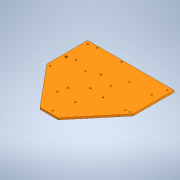
# Autodesk Inventor part: bp_v2
Saved by Autodesk Inventor 2020.3 (Build 243373000, 373)
## iProperties
Created: 2020-06-30
Part Number: bp_v2
Material: PET Plastic
Document SubType Name: Modeling
Designer: Devin
Density: 1.541 g/cm^3
Appearance: Orange
Author: Devin
Autodesk Inventor part; units mm, degrees
ref_plane "YZ Plane" through (0, 0, 0) normal (1, 0, 0) x (0, 1, 0)
ref_plane "XZ Plane" through (0, 0, 0) normal (0, 1, 0) x (-1, 0, 0)
ref_plane "XY Plane" through (0, 0, 0) normal (0, 0, 1) x (1, 0, 0)
sketch "Sketch1" plane through (0, 0, 0) normal (0, 1, 0) x (-1, 0, 0)
  line L0 (0, 0) -> (-190, 0)
  line L1 (-95, 180) -> (-75, 180)
  line L2 (-75, 180) -> (0, 90)
  line L3 (-95, 180) -> (-115, 180)
  line L4 (-115, 180) -> (-190, 90)
  line L5 (0, 0) -> (0, 90)
  line L6 (-190, 0) -> (-190, 90)
  dimension "d1" = 190
  dimension "d39" = 20
  dimension "d40" = 20
  constraints: 14 end point, 3 horizontal, 1 parallel, 1 vertical
  measures "d1" distance of L0.start L0.end
  measures "d39" distance of L1.start L1.end
  measures "d40" distance of L1.start L3.end
extrude "Extrusion1" add sketch "Sketch1" along normal blind 4
sketch "Sketch14" plane through (0, 4, 0) normal (0, 1, 0) x (1, 0, 0)
  line L0 (190, 0) -> (0, 0) projected
  line L1 (0, 0) -> (0, -7.5)
  line L2 (0, 0) -> (0, -15) projected
  line L3 (0, -90) -> (75, -180) projected
  circle A0 centre (7.5, -7.5) radius 1.55
  circle A1 centre (7.5, -90) radius 1.55
  line L4 (75, -180) -> (115, -180) projected
  circle A2 centre (182.5, -7.5) radius 1.55
  circle A3 centre (182.5, -90) radius 1.55
  circle A4 centre (95, -172.5) radius 1.55
  dimension "d68" = 7.5
  dimension "d71" = 3.1
  dimension "d72" = 3.1
  dimension "d74" = 3.1
  constraints: 5 centre point, 2 end point, 1 midpoint
  measures "d68" distance of L0.end L1.end
  measures "d71" diameter of A0
  measures "d72" diameter of A1
  measures "d74" diameter of A4
extrude "Extrusion10" cut sketch "Sketch14" against normal blind 10
sketch "Sketch17" plane through (0, 4, 0) normal (0, 1, 0) x (1, 0, 0)
  line L0 (93.28, -54.34) -> (12, -54.34)
  line L1 (12, -54.34) -> (12, -1)
  line L2 (12, -1) -> (93.28, -1)
  line L3 (93.28, -1) -> (93.28, -54.34)
  line L4 (93.28, -54.34) -> (93.28, -50.7586)
  circle A0 centre (79.5513, -50.7586) radius 1.55
  circle A1 centre (24.6238, -50.7586) radius 1.55
  line L5 (93.28, -1) -> (93.28, -3.8194)
  circle A2 centre (78.3321, -3.8194) radius 1.55
  circle A3 centre (24.6238, -3.8194) radius 1.55
  point P0 (0, 0)
  dimension "d101" = 81.28
  dimension "d102" = 53.34
  dimension "d106" = 3.1
  dimension "d107" = 3.1
  dimension "d111" = 3.1
  dimension "d112" = 3.1
  dimension "d113" = 14.9479
  dimension "d114" = 2.8194
  dimension "d115" = 12.6238
  dimension "d116" = 2.8194
  dimension "d117" = 12.6238
  dimension "d118" = 3.5814
  dimension "d119" = 3.5814
  dimension "d120" = 13.7287
  constraints: 12 end point, 4 centre point, 2 parallel, 2 point on line, 1 perpendicular
  measures "d101" distance of L0.start L0.end
  measures "d102" distance of L0.end L1.end
  measures "d106" diameter of A0
  measures "d107" diameter of A1
  measures "d111" diameter of A2
  measures "d112" diameter of A3
  measures "d113" distance from line of L3 A2.centre
  measures "d114" distance from line of L2 A2.centre
  measures "d115" distance from line of L1 A3.centre
  measures "d116" distance from line of L2 A3.centre
  measures "d117" distance from line of L1 A1.centre
  measures "d118" distance from line of L0 A1.centre
  measures "d119" distance from line of L0 A0.centre
  measures "d120" distance from line of L3 A0.centre
sketch "Sketch18" plane through (0, 4, 0) normal (0, 1, 0) x (1, 0, 0)
  line L0 (190, 0) -> (0, 0) projected
  line L1 (190, -90) -> (190, 0) projected
  line L2 (175, -10) -> (125, -10)
  line L3 (122, -13) -> (122, -92)
  line L4 (125, -95) -> (175, -95)
  line L5 (178, -92) -> (178, -13)
  circle A0 centre (174.5, -91.5) radius 1.375
  circle A1 centre (125.5, -91.5) radius 1.4481
  circle A2 centre (125.5, -33.5) radius 1.375
  circle A3 centre (174.5, -33.5) radius 1.375
  arc A4 (125, -10) -> (122, -13) centre (125, -13) ccw
  arc A5 (178, -13) -> (175, -10) centre (175, -13) ccw
  arc A6 (175, -95) -> (178, -92) centre (175, -92) ccw
  arc A7 (122, -92) -> (125, -95) centre (125, -92) ccw
  point P0 (122, -10)
  dimension "d129" = 2.75
  dimension "d130" = 3.5
  dimension "d131" = 3.5
  dimension "d132" = 49
  dimension "d133" = 3.5
  dimension "d134" = 2.75
  dimension "d135" = 3.5
  dimension "d136" = 58
  dimension "d137" = 2.75
  dimension "d138" = 3.5
  dimension "d139" = 49
  dimension "d140" = 3
  dimension "d141" = 3
  dimension "d142" = 3
  dimension "d143" = 3
  constraints: 8 centre point, 8 end point, 8 point on circle, 8 tangent, 2 parallel, 2 point on line, 1 perpendicular
  measures "d129" diameter of A0
  measures "d130" distance from line of A0.centre L4
  measures "d131" distance from line of A0.centre L5
  measures "d132" distance of A0.centre A1.centre
  measures "d133" distance from line of A1.centre L4
  measures "d134" diameter of A2
  measures "d135" distance from line of L3 A2.centre
  measures "d136" distance of A1.centre A2.centre
  measures "d137" diameter of A3
  measures "d138" distance from line of L5 A3.centre
  measures "d139" distance of A3.centre A2.centre
  measures "d140" radius of A4
  measures "d141" radius of A5
  measures "d142" radius of A6
  measures "d143" radius of A7
sketch "Sketch19" plane through (0, 4, 0) normal (0, 1, 0) x (1, 0, 0)
  line L0 (49.4722, -56.3802) -> (119.4722, -56.3802)
  line L1 (119.4722, -56.3802) -> (119.4722, -154.8802)
  line L2 (119.4722, -154.8802) -> (49.4722, -154.8802)
  line L3 (49.4722, -154.8802) -> (49.4722, -56.3802)
  circle A0 centre (56.4722, -61.3802) radius 1.375
  circle A1 centre (112.4722, -61.3802) radius 1.375
  circle A2 centre (104.4722, -131.2502) radius 1.375
  circle A3 centre (64.4722, -131.2502) radius 1.375
  point P0 (0, 0)
  dimension "d144" = 70
  dimension "d145" = 98.5
  dimension "d151" = 2.75
  dimension "d152" = 2.75
  dimension "d153" = 2.75
  dimension "d154" = 2.75
  dimension "d155" = 5
  dimension "d156" = 69.87
  dimension "d157" = 5
  dimension "d158" = 69.87
  dimension "d159" = 40
  dimension "d160" = 56
  constraints: 8 end point, 4 centre point, 2 parallel, 1 horizontal, 1 perpendicular
  measures "d144" distance of L0.start L0.end
  measures "d145" distance of L0.end L1.end
  measures "d151" diameter of A0
  measures "d152" diameter of A1
  measures "d153" diameter of A2
  measures "d154" diameter of A3
  measures "d155" distance from line of L0 A0.centre
  measures "d156" vertical distance of A3.centre A0.centre
  measures "d157" distance from line of L0 A1.centre
  measures "d158" vertical distance of A2.centre A1.centre
  measures "d159" distance of A2.centre A3.centre
  measures "d160" distance of A1.centre A0.centre
extrude "Extrusion13" cut sketch "Sketch17" against normal through all contours A0 | A1 | A2 | A3
extrude "Extrusion14" cut sketch "Sketch18" against normal through all contours A0 | A1 | A2 | A3
extrude "Extrusion15" cut sketch "Sketch19" against normal through all contours A0 | A1 | A2 | A3
sketch "Sketch22" plane through (0, 0, 0) normal (0, -1, 0) x (1, 0, 0)
  circle A0 centre (112.4722, 61.3802) radius 1.375 projected
  circle A1 centre (112.4722, 61.3802) radius 2.5
  circle A2 centre (56.4722, 61.3802) radius 1.375 projected
  circle A3 centre (56.4722, 61.3802) radius 2.5
  circle A4 centre (64.4722, 131.2502) radius 1.375 projected
  circle A5 centre (64.4722, 131.2502) radius 2.5
  circle A6 centre (104.4722, 131.2502) radius 1.375 projected
  circle A7 centre (104.4722, 131.2502) radius 2.5
  point P0 (0, 0)
  dimension "d171" = 5
  dimension "d172" = 5
  dimension "d173" = 5
  dimension "d174" = 5
  constraints: 4 centre point, 4 coincident
  measures "d171" diameter of A1
  measures "d172" diameter of A3
  measures "d173" diameter of A5
  measures "d174" diameter of A7
extrude "Extrusion16" cut sketch "Sketch22" against normal blind 2
sketch "Sketch23" plane through (0, 0, 0) normal (0, -1, 0) x (1, 0, 0)
  circle A0 centre (125.5, 33.5) radius 1.375 projected
  circle A1 centre (125.5, 91.5) radius 1.4481 projected
  circle A2 centre (174.5, 91.5) radius 1.375 projected
  circle A3 centre (174.5, 33.5) radius 1.375 projected
  line L0 (174.5, 30.3) -> (171.7287, 31.9)
  line L1 (171.7287, 31.9) -> (171.7287, 35.1)
  line L2 (171.7287, 35.1) -> (174.5, 36.7)
  line L3 (174.5, 36.7) -> (177.2713, 35.1)
  line L4 (177.2713, 35.1) -> (177.2713, 31.9)
  line L5 (177.2713, 31.9) -> (174.5, 30.3)
  line L6 (125.5, 30.3) -> (122.7287, 31.9)
  line L7 (122.7287, 31.9) -> (122.7287, 35.1)
  line L8 (122.7287, 35.1) -> (125.5, 36.7)
  line L9 (125.5, 36.7) -> (128.2713, 35.1)
  line L10 (128.2713, 35.1) -> (128.2713, 31.9)
  line L11 (128.2713, 31.9) -> (125.5, 30.3)
  line L12 (125.5, 88.3) -> (122.7287, 89.9)
  line L13 (122.7287, 89.9) -> (122.7287, 93.1)
  line L14 (122.7287, 93.1) -> (125.5, 94.7)
  line L15 (125.5, 94.7) -> (128.2713, 93.1)
  line L16 (128.2713, 93.1) -> (128.2713, 89.9)
  line L17 (128.2713, 89.9) -> (125.5, 88.3)
  line L18 (174.5, 88.3) -> (171.7287, 89.9)
  line L19 (171.7287, 89.9) -> (171.7287, 93.1)
  line L20 (171.7287, 93.1) -> (174.5, 94.7)
  line L21 (174.5, 94.7) -> (177.2713, 93.1)
  line L22 (177.2713, 93.1) -> (177.2713, 89.9)
  line L23 (177.2713, 89.9) -> (174.5, 88.3)
  circle A4 centre (78.3321, 3.8194) radius 1.55 projected
  circle A5 centre (79.5513, 50.7586) radius 1.55 projected
  circle A6 centre (24.6238, 50.7586) radius 1.55 projected
  circle A7 centre (24.6238, 3.8194) radius 1.55 projected
  line L24 (78.3321, 0.5194) -> (75.4742, 2.1694)
  line L25 (75.4742, 2.1694) -> (75.4742, 5.4694)
  line L26 (75.4742, 5.4694) -> (78.3321, 7.1194)
  line L27 (78.3321, 7.1194) -> (81.19, 5.4694)
  line L28 (81.19, 5.4694) -> (81.19, 2.1694)
  line L29 (81.19, 2.1694) -> (78.3321, 0.5194)
  line L30 (24.6238, 0.5194) -> (21.7659, 2.1694)
  line L31 (21.7659, 2.1694) -> (21.7659, 5.4694)
  line L32 (21.7659, 5.4694) -> (24.6238, 7.1194)
  line L33 (24.6238, 7.1194) -> (27.4817, 5.4694)
  line L34 (27.4817, 5.4694) -> (27.4817, 2.1694)
  line L35 (27.4817, 2.1694) -> (24.6238, 0.5194)
  line L36 (79.5513, 47.4586) -> (76.6934, 49.1086)
  line L37 (76.6934, 49.1086) -> (76.6934, 52.4086)
  line L38 (76.6934, 52.4086) -> (79.5513, 54.0586)
  line L39 (79.5513, 54.0586) -> (82.4092, 52.4086)
  line L40 (82.4092, 52.4086) -> (82.4092, 49.1086)
  line L41 (82.4092, 49.1086) -> (79.5513, 47.4586)
  line L42 (24.6238, 47.4586) -> (21.7659, 49.1086)
  line L43 (21.7659, 49.1086) -> (21.7659, 52.4086)
  line L44 (21.7659, 52.4086) -> (24.6238, 54.0586)
  line L45 (24.6238, 54.0586) -> (27.4817, 52.4086)
  line L46 (27.4817, 52.4086) -> (27.4817, 49.1086)
  line L47 (27.4817, 49.1086) -> (24.6238, 47.4586)
  point P0 (0, 0)
  constraints: 96 end point, 8 coincident, 104 other
extrude "Extrusion17" cut sketch "Sketch23" against normal blind 2 contours A0 | A1 | A2 | A3 | L0 L1 L2 L3 L4 L5 | L6 L7 L8 L9 L10 L11 | L12 L13 L14 L15 L16 L17 | L18 L19 L20 L21 L22 L23 | A4 | A5 | L24 L25 L26 L27 L28 L29 | L30 L31 L32 L33 L34 L35 | L36 L37 L38 L39 L40 L41 | L42 L43 L44 L45 L46 L47
sketch "Sketch24" plane through (0, 4, 0) normal (0, 1, 0) x (1, 0, 0)
  circle A0 centre (56.4722, -61.3802) radius 2.5 projected
  circle A1 centre (93.9722, -88.3552) radius 1.55
  circle A2 centre (68.9722, -112.4052) radius 1.55
  point P0 (0, 0)
  dimension "d206" = 3.1
  dimension "d208" = 3.1
  dimension "d209" = 25
  dimension "d210" = 24.05
  constraints: 2 centre point
  measures "d206" diameter of A1
  measures "d208" diameter of A2
  measures "d209" horizontal distance of A2.centre A1.centre
  measures "d210" vertical distance of A2.centre A1.centre
extrude "Extrusion18" cut sketch "Sketch24" against normal blind 10 contours A1 | A2
sketch "Sketch25" plane through (0, 4, 0) normal (0, 1, 0) x (1, 0, 0)
  circle A0 centre (7.5, -90) radius 1.55 projected
  circle A1 centre (7.5, -55) radius 2.5
  point P0 (0, 0)
  dimension "d202" = 5
  constraints: 1 centre point
  measures "d202" diameter of A1
extrude "Extrusion19" cut sketch "Sketch25" against normal blind 10 contours A1
sketch "Sketch26" plane through (0, 0, 0) normal (0, -1, 0) x (1, 0, 0)
  circle A0 centre (93.9722, 88.3552) radius 1.55 projected
  circle A1 centre (93.9722, 88.3552) radius 2.5
  circle A2 centre (68.9722, 112.4052) radius 1.55 projected
  circle A3 centre (68.9722, 112.4052) radius 2.5
  point P0 (0, 0)
  dimension "d211" = 5
  dimension "d212" = 5
  constraints: 2 centre point, 2 coincident
  measures "d211" diameter of A1
  measures "d212" diameter of A3
extrude "Extrusion20" cut sketch "Sketch26" against normal blind 2
body "Solid1"
